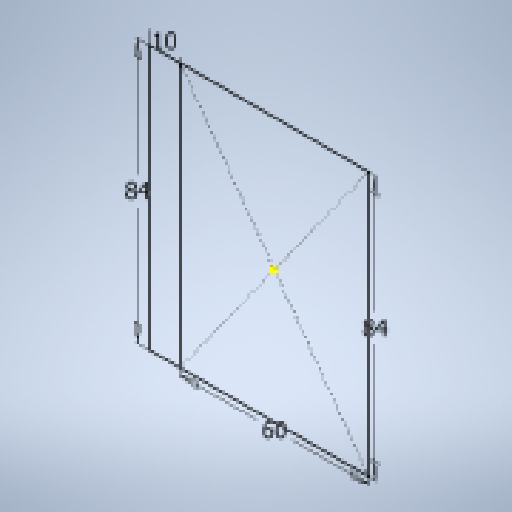
# Autodesk Inventor part: power_board
Saved by Autodesk Inventor 2025 (Build 290162000, 162)
## iProperties
Created: 2026-08-11
Part Number: power_board
Material: Типовые
Document SubType Name: Modeling
Designer: garin
Density: 1 g/cm^3
Appearance: По умолчанию
Author: garin
Autodesk Inventor part; units mm, degrees
ref_plane "YZ Plane" through (0, 0, 0) normal (1, 0, 0) x (0, 1, 0)
ref_plane "XZ Plane" through (0, 0, 0) normal (0, 1, 0) x (-1, 0, 0)
ref_plane "XY Plane" through (0, 0, 0) normal (0, 0, 1) x (1, 0, 0)
sketch "Эскиз1" plane through (0, 0, 0) normal (0, 0, 1) x (1, 0, 0)
  line L0 (-30, 41.5) -> (26, 41.5)
  line L1 (30, 37.5) -> (30, -37.5)
  line L2 (26, -41.5) -> (-30, -41.5)
  line L3 (-30, -41.5) -> (-30, 41.5)
  line L4 (-30, 41.5) -> (30, -41.5) construction
  line L5 (30, 41.5) -> (-30, -41.5) construction
  line L6 (-30, -41.5) -> (-41, -41.5)
  line L7 (-45, -37.5) -> (-45, 37.5)
  line L8 (-41, 41.5) -> (-30, 41.5)
  line L9 (-30, 41.5) -> (-30, -41.5)
  line L10 (-41, -41.5) -> (-45, -37.5)
  line L11 (-45, 37.5) -> (-41, 41.5)
  line L12 (26, 41.5) -> (30, 37.5)
  line L13 (26, -41.5) -> (30, -37.5)
  point P0 (0, 0)
  point P1 (-45, 41.5)
  point P2 (-45, -41.5)
  dimension "d0" = 60
  dimension "d1" = 83
  dimension "d2" = 15
  dimension "d3" = 83
  dimension "d6" = 4
  dimension "d7" = 4
  dimension "d8" = 4
  dimension "d9" = 4
  dimension "d10" = 4
  dimension "d11" = 4
  dimension "d12" = 4
  dimension "d13" = 4
  constraints: 28 end point, 8 point on line, 4 parallel, 2 horizontal, 2 midpoint, 2 perpendicular
  measures "d0" distance of L4.end L2.end
  measures "d1" distance of L5.start L4.end
  measures "d2" distance of point (-45, 41.5) L8.end
  measures "d3" distance of point (-45, -41.5) point (-45, 41.5)
  measures "d6" distance of L6.end point (-45, -41.5)
  measures "d7" distance of L7.start point (-45, -41.5)
  measures "d8" distance of L7.end point (-45, 41.5)
  measures "d9" distance of L8.start point (-45, 41.5)
  measures "d10" distance of L0.end L5.start
  measures "d11" distance of L1.start L5.start
  measures "d12" distance of L2.start L4.end
  measures "d13" distance of L1.end L4.end
extrude "Выдавливание1" add sketch "Эскиз1" along normal blind 1.5
equation "\"d7\" = d6"
equation "\"d9\" = d8"
equation "\"d10\" = d6"
equation "\"d11\" = d10"
